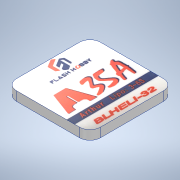
# Autodesk Inventor part: Heatsink
Saved by Autodesk Inventor 2022 (Build 260153000, 153)
## iProperties
Created: 2022-09-17
Part Number: Heatsink
Material: Aluminum 6061
Document SubType Name: Modeling
Designer: Nathan Cai
Density: 2.7 g/cm^3
Appearance: Aluminum - Flat
Author: Nathan Cai
Autodesk Inventor part; units mm, degrees
ref_plane "YZ Plane" through (0, 0, 0) normal (1, 0, 0) x (0, 1, 0)
ref_plane "XZ Plane" through (0, 0, 0) normal (0, 1, 0) x (-1, 0, 0)
ref_plane "XY Plane" through (0, 0, 0) normal (0, 0, 1) x (1, 0, 0)
sketch "Sketch1" plane through (0, 0, 0) normal (0, 1, 0) x (-1, 0, 0)
  line L0 (-8, 8) -> (8, 8)
  line L1 (8, 8) -> (8, -8)
  line L2 (8, -8) -> (-8, -8)
  line L3 (-8, -8) -> (-8, 8)
  line L4 (-8, 8) -> (8, -8) construction
  line L5 (8, 8) -> (-8, -8) construction
  point P0 (0, 0)
  dimension "d0" = 16
  dimension "d1" = 16
  constraints: 12 end point, 2 midpoint, 2 parallel, 1 horizontal, 1 perpendicular
  measures "d0" distance of L1.end L2.end
  measures "d1" distance of L0.end L1.end
extrude "Extrusion1" add sketch "Sketch1" along normal blind 1.75
fillet "Fillet1" radius 2 4 edges at (-8, 0.875, 8) (8, 0.875, 8) (8, 0.875, -8) (-8, 0.875, -8)
sketch "Sketch2" plane through (0, 1.75, 0) normal (0, 1, 0) x (1, 0, 0)
  line L0 (-8, 8) -> (8, 8) construction
  line L1 (8, 8) -> (8, -8) construction
  line L2 (8, -8) -> (-8, -8) construction
  line L3 (-8, -8) -> (-8, 8) construction
  line L4 (6, 8) -> (-6, 8) projected
  line L5 (-8, 6) -> (-8, -6) projected
  line L6 (8, -6) -> (8, 6) projected
  point P0 (0, 0)
  constraints: 3 point on line, 1 collinear, 2 other
decal "Decal1"
body "Solid1"
